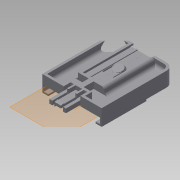
# Autodesk Inventor part: Wanne
Saved by Autodesk Inventor 2015 (Build 190159000, 159)
## iProperties
Created: 2016-03-30
Part Number: Wanne
Material: Generisch
Document SubType Name: Modeling
Designer: Bene
Density: 1 g/cm^3
Appearance: Vorgabe
Author: Bene
Autodesk Inventor part; units mm, degrees
ref_plane "YZ Plane" through (0, 0, 0) normal (1, 0, 0) x (0, 1, 0)
ref_plane "XZ Plane" through (0, 0, 0) normal (0, 1, 0) x (-1, 0, 0)
sketch "Skizze1" plane through (0, 0, 0) normal (0, 0, 1) x (1, 0, 0)
  spline S0 degree 3 poles (-32.4027, 58.6038) (-32.4242, 58.2127) (-32.4349, 57.8189) (-32.4464, 57.0431) (-32.4479, 56.5998) (-32.4483, 56.24) knots 0 0 0 0 0.502492 0.502492 1 1 1 1
  spline S1 degree 3 poles (-20.1386, 68.0766) (-22.3806, 68.0766) (-24.2323, 68.0757) (-27.4543, 67.1708) (-28.3503, 66.6459) (-29.5894, 65.7879) (-30.2592, 65.1575) (-31.2004, 63.6796) (-31.6677, 62.8135) (-32.3154, 60.3747) (-32.41, 59.3008) (-32.4496, 58.5318) knots 0 0 0 0 0.672578 0.672578 1.163557 1.163557 1.787429 1.787429 2.153382 2.153382 2.479485 2.479485 2.479485 2.479485
  line L0 (20.1262, 68.08) -> (-20.1416, 68.08)
  spline S2 degree 3 poles (32.4493, 58.5386) (32.4116, 59.2663) (32.3242, 60.2689) (31.7597, 62.5356) (31.3605, 63.3619) (30.4007, 65.0232) (29.6947, 65.6721) (28.4754, 66.5948) (27.6054, 67.0699) (24.5181, 68.0769) (22.4773, 68.0766) (20.1224, 68.0766) knots 0 0 0 0 0.218603 0.218603 0.458625 0.458625 0.933122 0.933122 1.531383 1.531383 2.646416 2.646416 2.646416 2.646416
  spline S3 degree 3 poles (32.4483, 56.2387) (32.4479, 56.5985) (32.4464, 57.0427) (32.435, 57.8141) (32.4245, 58.2022) (32.4036, 58.5883) knots 0 0 0 0 0.500631 0.500631 1 1 1 1
  line L1 (32.4484, 56.24) -> (32.4914, 56.24)
  spline S4 degree 3 poles (32.4916, 55.7088) (32.4916, 55.8023) (32.4916, 55.8867) (32.4915, 56.0637) (32.4915, 56.1519) (32.4914, 56.24) knots 0 0 0 0 0.502221 0.502221 1 1 1 1
  line L2 (32.495, -55.7116) -> (32.495, 55.7118)
  spline S5 degree 3 poles (32.4914, -56.24) (32.4915, -56.1518) (32.4915, -56.0635) (32.4916, -55.8863) (32.4916, -55.7993) (32.4916, -55.7082) knots 0 0 0 0 0.497816 0.497816 1 1 1 1
  line L3 (32.4483, -56.24) -> (32.4914, -56.24)
  spline S6 degree 3 poles (32.4036, -58.5883) (32.4245, -58.2023) (32.435, -57.8137) (32.4464, -57.0431) (32.4479, -56.5998) (32.4483, -56.24) knots 0 0 0 0 0.499187 0.499187 1 1 1 1
  spline S7 degree 3 poles (20.1238, -68.0766) (22.37, -68.0766) (24.2191, -68.0767) (27.4415, -67.1764) (28.3392, -66.6524) (29.5878, -65.7904) (30.256, -65.1597) (31.1955, -63.6888) (31.6649, -62.8216) (32.3151, -60.3783) (32.4099, -59.3023) (32.4496, -58.5321) knots 0 0 0 0 0.673858 0.673858 1.166886 1.166886 1.797679 1.797679 2.170612 2.170612 2.502894 2.502894 2.502894 2.502894
  line L4 (-20.1262, -68.08) -> (20.1267, -68.08)
  spline S8 degree 3 poles (-32.4488, -58.5488) (-32.4087, -59.3142) (-32.3134, -60.3877) (-31.6647, -62.8189) (-31.1986, -63.684) (-30.2648, -65.1459) (-29.6029, -65.78) (-28.3413, -66.651) (-27.4446, -67.175) (-24.2213, -68.0768) (-22.3702, -68.0766) (-20.1233, -68.0766) knots 0 0 0 0 0.22994 0.22994 0.486349 0.486349 0.910106 0.910106 1.233054 1.233054 1.675094 1.675094 1.675094 1.675094
  spline S9 degree 3 poles (-32.4483, -56.2387) (-32.4479, -56.5985) (-32.4464, -57.0427) (-32.435, -57.8141) (-32.4245, -58.2022) (-32.4036, -58.5883) knots 0 0 0 0 0.500631 0.500631 1 1 1 1
  line L5 (-32.4484, -56.24) -> (-32.4914, -56.24)
  spline S10 degree 3 poles (-32.4916, -55.7088) (-32.4916, -55.8023) (-32.4916, -55.8867) (-32.4915, -56.0637) (-32.4915, -56.1519) (-32.4914, -56.24) knots 0 0 0 0 0.502221 0.502221 1 1 1 1
  line L6 (-32.495, 55.7116) -> (-32.495, -55.7118)
  spline S11 degree 3 poles (-32.4914, 56.24) (-32.4915, 56.1518) (-32.4915, 56.0635) (-32.4916, 55.8863) (-32.4916, 55.7993) (-32.4916, 55.7082) knots 0 0 0 0 0.497816 0.497816 1 1 1 1
  line L7 (-32.4483, 56.24) -> (-32.4914, 56.24)
  line L8 (11, -17.58) -> (-11, -17.58)
  line L9 (-11, -17.58) -> (-11, -68.08)
  line L10 (-11, -68.08) -> (11, -68.08)
  line L11 (11, -68.08) -> (11, -17.58)
  line L12 (0, -17.58) -> (36.495, -17.58)
  line L13 (36.495, -17.58) -> (36.495, 62.08)
  line L14 (27.495, 71.08) -> (0, 71.08)
  line L15 (0, 71.08) -> (0, -17.58)
  line L16 (20.1263, 68.08) -> (-20.1435, 68.08)
  arc A0 (36.495, 62.08) -> (27.495, 71.08) centre (27.495, 62.08) ccw
  line L17 (-0.0077, 79.9624) -> (-0.0077, -73.7985)
  line L18 (-20.1416, 68.08) -> (20.1262, 68.08)
  spline S12 degree 3 poles (-32.4646, 58.5386) (-32.4269, 59.2663) (-32.3395, 60.2689) (-31.775, 62.5356) (-31.3758, 63.3619) (-30.416, 65.0232) (-29.7101, 65.6721) (-28.4907, 66.5948) (-27.6207, 67.0699) (-24.5335, 68.0769) (-22.4926, 68.0766) (-20.1378, 68.0766) knots 0 0 0 0 0.218603 0.218603 0.458625 0.458625 0.933122 0.933122 1.531383 1.531383 2.646416 2.646416 2.646416 2.646416
  spline S13 degree 3 poles (-32.4637, 56.2387) (-32.4633, 56.5985) (-32.4618, 57.0427) (-32.4504, 57.8141) (-32.4399, 58.2022) (-32.4189, 58.5883) knots 0 0 0 0 0.500631 0.500631 1 1 1 1
  line L19 (-32.4638, 56.24) -> (-32.5067, 56.24)
  spline S14 degree 3 poles (-32.5069, 55.7088) (-32.5069, 55.8023) (-32.5069, 55.8867) (-32.5069, 56.0637) (-32.5068, 56.1519) (-32.5067, 56.24) knots 0 0 0 0 0.502221 0.502221 1 1 1 1
  line L20 (-32.5104, -55.7116) -> (-32.5104, 55.7118)
  line L21 (-11.0154, -17.58) -> (10.9846, -17.58)
  line L22 (-11.0154, -68.08) -> (-11.0154, -17.58)
  line L23 (-0.0154, -17.58) -> (-36.5104, -17.58)
  line L24 (-36.5104, -17.58) -> (-36.5104, 62.08)
  line L25 (-27.5104, 71.08) -> (-0.0154, 71.08)
  line L26 (-0.0154, 71.08) -> (-0.0154, -17.58)
  line L27 (-20.1417, 68.08) -> (20.1281, 68.08)
  arc A1 (-27.5104, 71.08) -> (-36.5104, 62.08) centre (-27.5104, 62.08) ccw
  point P0 (0, 0)
  point P1 (-0.0154, 0)
  dimension "d0" = 3
  dimension "d1" = 4
  dimension "d2" = 9
  constraints: 22 symmetric about line, 18 end point, 4 point on circle, 2 centre point, 2 parallel, 2 tangent, 1 horizontal, 1 midpoint, 1 perpendicular, 1 vertical, 1 other
  measures "d0" distance between parallel lines of L14 L16
  measures "d1" distance between parallel lines of L13 L2
  measures "d2" radius of A0
extrude "Extrusion1" add sketch "Skizze1" along normal blind 3 contours L15 L14 A0 L13 L12 L8 | L26 L8 L21 L23 L24 A1 L25
ref_plane "Arbeitsebene1" through (0, 0, 0) normal (0, 0, 1) x (1, 0, 0)
ref_plane "Arbeitsebene2" through (-10.5, -17.58, 1.25) normal (0, 0, 1) x (1, 0, 0)
sketch "Skizze2" plane through (-10.5, -17.58, 1.25) normal (0, 0, 1) x (1, 0, 0)
  line L0 (21.5, 0) -> (-0.5, 0) projected
  line L1 (-0.5, 0) -> (-0.5, -50.5) projected
  line L2 (-0.5, -50.5) -> (21.5, -50.5) projected
  line L3 (21.5, -50.5) -> (21.5, 0) projected
  line L4 (0, 0) -> (21, 0) projected
  line L5 (0, 0) -> (0, -17.5) projected
  line L6 (0, -17.5) -> (21, -17.5) projected
  line L7 (21, 0) -> (21, -17.5) projected
  line L8 (20.6414, -17.5) -> (16.6414, -17.5)
  line L9 (16.6414, -17.5) -> (16.6414, 8.5)
  line L10 (16.6414, 8.5) -> (20.6414, 8.5)
  line L11 (20.6414, 8.5) -> (20.6414, -17.5)
  line L12 (10.5, -17.5) -> (14.5, -17.5)
  line L13 (14.5, -17.5) -> (14.5, 8.5)
  line L14 (14.5, 8.5) -> (10.5, 8.5)
  line L15 (10.5, 8.5) -> (10.5, -17.5)
  line L16 (10.5, -21.3506) -> (10.5, 17.58)
  line L17 (-0.5, 0) -> (21.5, 0)
  line L18 (21, 0) -> (0, 0)
  line L19 (0, 0) -> (0, -17.5)
  line L20 (0.3587, -17.5) -> (4.3587, -17.5)
  line L21 (4.3587, -17.5) -> (4.3587, 8.5)
  line L22 (4.3587, 8.5) -> (0.3587, 8.5)
  line L23 (0.3587, 8.5) -> (0.3587, -17.5)
  line L24 (10.5, -17.5) -> (6.5, -17.5)
  line L25 (6.5, -17.5) -> (6.5, 8.5)
  line L26 (6.5, 8.5) -> (10.5, 8.5)
  line L27 (10.5, 8.5) -> (10.5, -17.5)
  dimension "d5" = 4
  dimension "d6" = 26
  dimension "d7" = 4
  constraints: 34 end point, 13 symmetric about line, 4 parallel, 3 point on line, 2 horizontal, 2 perpendicular, 1 midpoint, 1 vertical
  measures "d5" distance of L9.end L10.end
  measures "d6" distance of L8.end L9.end
  measures "d7" distance of L14.end L13.end
extrude "Extrusion2" add sketch "Skizze2" along normal blind 5 contours L11 L6 L9 L0 | L0 L9 L10 L11 | L13 L6 L15 L0 | L0 L15 L14 L13 | L15 L6 L25 L0 | L0 L25 L26 L15 | L23 L22 L21 L0 | L0 L21 L6 L23
sketch "Skizze3" plane through (4, -35.08, 1.25) normal (1, 0, 0) x (0, 0, -1)
  line L0 (-1.75, 26) -> (-1.75, 17.5) projected
  line L1 (-1.75, 26) -> (-5, 26) projected
  line L2 (-5, 0) -> (-5, 26) projected
  line L3 (0, 0) -> (-5, 0) projected
  line L4 (0, 0) -> (0, 17.5) projected
  line L5 (-1.75, 17.5) -> (0, 17.5) projected
  line L6 (-5, 0) -> (-5.747, 3.8675)
  line L7 (-5.747, 3.8675) -> (-5, 3.8675)
  point P0 (1.25, 35.08)
  constraints: 4 end point, 1 perpendicular, 1 point on line
extrude "Extrusion3" add sketch "Skizze3" against normal up to surface (8 mm away) contours L2 L6 L7
sketch "Skizze4" plane through (-4, -35.08, 1.25) normal (0, -1, 0) x (1, 0, 0)
  line L0 (-6.5, 0) -> (14.5, 0) projected
  line L1 (-6.5, 5.5) -> (-6.5, 0) projected
  line L2 (14.5, 5.5) -> (-6.5, 5.5) projected
  line L3 (14.5, 0) -> (14.5, 5.5) projected
  line L4 (8, 0) -> (8, 5) projected
  line L5 (0.1003, 0) -> (8, 0)
  line L6 (8, 0) -> (8, 1.8913)
  line L7 (8, 1.8913) -> (0.1003, 1.8913)
  line L8 (0.1003, 1.8913) -> (0.1003, 0)
  point P0 (4, -1.25)
  constraints: 8 end point, 2 parallel, 2 point on line, 1 horizontal, 1 perpendicular
extrude "Extrusion4" cut sketch "Skizze4" against normal up to surface (17.5 mm away) contours L8 L7 L4 L0
ref_plane "Arbeitsebene3" through (-29.2488, -52.025, -6.9) normal (0, 0, -1) x (0, 1, 0)
sketch "Skizze5" plane through (0, 0, 0) normal (0, 0, -1) x (-1, 0, 0)
  line L0 (36.5104, -17.58) -> (0.0154, -17.58) projected
  line L1 (36.5104, 62.08) -> (36.5104, -17.58) projected
  arc A0 (36.5104, 62.08) -> (27.5104, 71.08) centre (27.5104, 62.08) ccw projected
  line L2 (0.0154, 71.08) -> (27.5104, 71.08) projected
  line L3 (0.0154, -17.58) -> (0.0154, 71.08) projected
  line L4 (0, -17.58) -> (-36.495, -17.58) projected
  line L5 (0, 71.08) -> (0, -17.58) projected
  line L6 (-27.495, 71.08) -> (0, 71.08) projected
  arc A1 (-27.495, 71.08) -> (-36.495, 62.08) centre (-27.495, 62.08) ccw projected
  line L7 (-36.495, -17.58) -> (-36.495, 62.08) projected
  line L8 (34.6104, -15.68) -> (1.9154, -15.68)
  line L9 (1.9154, -15.68) -> (1.9154, 69.18)
  line L10 (1.9154, 69.18) -> (27.5104, 69.18)
  arc A2 (34.6104, 62.08) -> (27.5104, 69.18) centre (27.5104, 62.08) ccw
  line L11 (34.6104, 62.08) -> (34.6104, -15.68)
  arc A3 (-27.495, 69.18) -> (-34.595, 62.08) centre (-27.495, 62.08) ccw
  line L12 (-27.495, 69.18) -> (-1.9, 69.18)
  line L13 (-1.9, 69.18) -> (-1.9, -15.68)
  line L14 (-1.9, -15.68) -> (-34.595, -15.68)
  line L15 (-34.595, -15.68) -> (-34.595, 62.08)
  line L16 (1.9154, -15.68) -> (-1.9, -15.68)
  line L17 (1.9154, 69.18) -> (-1.9, 69.18)
  line L18 (34.6104, -15.68) -> (34.6104, -17.58)
  line L19 (-34.595, -15.68) -> (-34.595, -17.58)
  point P0 (0, 0)
  dimension "d14" = 1.9
  dimension "d15" = 1.9
  constraints: 24 end point, 8 coincident, 4 point on circle, 2 centre point, 2 point on line, 1 parallel, 1 perpendicular, 8 other
  measures "d14" distance between parallel lines of L1 L11
  measures "d15" distance between parallel lines of L7 L15
extrude "Extrusion5" add sketch "Skizze5" along normal up to surface (6.9 mm away) contours L0 L18 L11 A2 L10 L17 L3 L2 A0 L1 | L0 L3 L16 L8 L18 | L3 L17 L9 L16 | L16 L13 L17 L5 | L5 L4 L19 L14 L16 | L17 L12 A3 L15 L19 L4 L7 A1 L6 L5
sketch "Skizze6" plane through (36.495, -17.58, -6.9) normal (0, 0, -1) x (-1, 0, 0)
  line L0 (38.4104, 1.9) -> (71.1054, 1.9) projected
  line L1 (38.4104, 86.76) -> (38.4104, 1.9) projected
  line L2 (64.0054, 86.76) -> (38.4104, 86.76) projected
  arc A0 (71.1054, 79.66) -> (64.0054, 86.76) centre (64.0054, 79.66) ccw projected
  line L3 (71.1054, 1.9) -> (71.1054, 79.66) projected
  line L4 (36.5104, 0) -> (36.5104, 88.66) projected
  line L5 (73.0054, 0) -> (36.5104, 0) projected
  line L6 (73.0054, 79.66) -> (73.0054, 0) projected
  arc A1 (73.0054, 79.66) -> (64.0054, 88.66) centre (64.0054, 79.66) ccw projected
  line L7 (36.5104, 88.66) -> (64.0054, 88.66) projected
  line L8 (0, 0) -> (0, 79.66) projected
  line L9 (36.495, 0) -> (0, 0) projected
  line L10 (36.495, 88.66) -> (36.495, 0) projected
  line L11 (9, 88.66) -> (36.495, 88.66) projected
  arc A2 (9, 88.66) -> (0, 79.66) centre (9, 79.66) ccw projected
  line L12 (1.9, 1.9) -> (34.595, 1.9) projected
  line L13 (1.9, 79.66) -> (1.9, 1.9) projected
  arc A3 (9, 86.76) -> (1.9, 79.66) centre (9, 79.66) ccw projected
  line L14 (34.595, 86.76) -> (9, 86.76) projected
  line L15 (34.595, 1.9) -> (34.595, 86.76) projected
  line L16 (73.0054, 0) -> (46.6364, 0) projected
  line L17 (71.1054, 0) -> (1.9, 0)
  line L18 (1.9, 0) -> (1.9, 76.76)
  line L19 (11.9, 86.76) -> (61.1054, 86.76)
  line L20 (71.1054, 76.76) -> (71.1054, 0)
  arc A4 (71.1054, 76.76) -> (61.1054, 86.76) centre (61.1054, 76.76) ccw
  arc A5 (11.9, 86.76) -> (1.9, 76.76) centre (11.9, 76.76) ccw
  point P0 (36.495, 17.58)
  dimension "d18" = 10
  constraints: 8 end point, 4 point on circle, 4 tangent, 2 centre point, 2 parallel, 1 equal radius, 1 horizontal, 1 perpendicular, 1 point on line
  measures "d18" radius of A4
extrude "Extrusion6" cut sketch "Skizze6" against normal up to surface (6.9 mm away) contours L1 L2 A4 L3 L0 | L0 L20 L5 L4 L19 L1 | A4 L2 A0 L3 | L4 L17 L10 L19 | L10 L9 L18 L12 L15 L19 | L15 L12 L13 A5 L14
sketch "Skizze7" plane through (-0.0154, 71.08, -6.9) normal (0, 0, -1) x (-1, 0, 0)
  line L0 (34.595, -9) -> (34.595, -88.66) projected
  line L1 (34.595, -9) -> (34.595, -88.66) projected
  line L2 (36.495, -88.66) -> (34.595, -88.66) projected
  line L3 (36.495, -9) -> (36.495, -88.66) projected
  arc A0 (36.495, -9) -> (27.495, 0) centre (27.495, -9) ccw projected
  line L4 (0, 0) -> (27.495, 0) projected
  line L5 (0, -1.9) -> (0, 0) projected
  line L6 (0, -1.9) -> (27.495, -1.9) projected
  arc A1 (34.595, -9) -> (27.495, -1.9) centre (27.495, -9) ccw projected
  line L7 (-34.6104, -88.66) -> (-34.6104, -9) projected
  arc A2 (-27.5104, -1.9) -> (-34.6104, -9) centre (-27.5104, -9) ccw projected
  line L8 (-0.0153, -1.9) -> (-27.5104, -1.9) projected
  line L9 (-0.0153, 0) -> (-0.0153, -1.9) projected
  line L10 (-27.5104, 0) -> (-0.0153, 0) projected
  arc A3 (-27.5104, 0) -> (-36.5104, -9) centre (-27.5104, -9) ccw projected
  line L11 (-36.5104, -88.66) -> (-36.5104, -9) projected
  line L12 (-34.6104, -88.66) -> (-36.5104, -88.66) projected
  line L13 (36.495, -88.66) -> (28.995, -88.66)
  line L14 (28.995, -88.66) -> (28.995, -33.66)
  line L15 (28.995, -33.66) -> (36.495, -33.66)
  line L16 (36.495, -33.66) -> (36.495, -88.66)
  line L17 (-36.5104, -88.66) -> (-29.0104, -88.66)
  line L18 (-29.0104, -88.66) -> (-29.0104, -33.66)
  line L19 (-29.0104, -33.66) -> (-36.5104, -33.66)
  line L20 (-36.5104, -33.66) -> (-36.5104, -88.66)
  point P0 (-0.0154, -71.08)
  dimension "d21" = 7.5
  dimension "d22" = 55
  dimension "d23" = 7.5
  constraints: 16 end point, 4 parallel, 2 horizontal, 2 perpendicular, 1 point on line
  measures "d21" distance of L14.end L15.end
  measures "d22" distance of L13.end L14.end
  measures "d23" distance of L19.end L18.end
extrude "Extrusion7" add sketch "Skizze7" along normal blind 2 contours L15 L3 L2 L0 | L0 L13 L14 L15 | L12 L11 L19 L7 | L7 L19 L18 L17
sketch "Skizze8" plane through (0, 0, 3) normal (0, 0, 1) x (1, 0, 0)
  line L0 (0, -9.08) -> (4, -9.08) projected
  line L1 (4, -9.08) -> (4, -17.58) projected
  line L2 (4, -17.58) -> (6.1414, -17.58) projected
  line L3 (6.1414, -17.58) -> (6.1414, -9.08) projected
  line L4 (6.1414, -9.08) -> (10.1414, -9.08) projected
  line L5 (10.1414, -9.08) -> (10.1414, -17.58) projected
  line L6 (10.1414, -17.58) -> (36.495, -17.58) projected
  line L7 (36.495, -17.58) -> (36.495, 62.08) projected
  arc A0 (36.495, 62.08) -> (27.495, 71.08) centre (27.495, 62.08) ccw projected
  line L8 (27.495, 71.08) -> (0, 71.08) projected
  line L9 (0, 71.08) -> (0, -9.08) projected
  line L10 (-10.1414, -17.58) -> (-10.1414, -9.08) projected
  line L11 (-10.1414, -9.08) -> (-6.1414, -9.08) projected
  line L12 (-6.1414, -9.08) -> (-6.1414, -17.58) projected
  line L13 (-6.1414, -17.58) -> (-4, -17.58) projected
  line L14 (-4, -17.58) -> (-4, -9.08) projected
  line L15 (-4, -9.08) -> (-0.0154, -9.08) projected
  line L16 (-0.0154, -9.08) -> (-0.0154, 71.08) projected
  line L17 (-0.0154, 71.08) -> (-27.5104, 71.08) projected
  arc A1 (-27.5104, 71.08) -> (-36.5104, 62.08) centre (-27.5104, 62.08) ccw projected
  line L18 (-36.5104, 62.08) -> (-36.5104, -17.58) projected
  line L19 (-36.5104, -17.58) -> (-10.1414, -17.58) projected
  point P0 (0, 0)
extrude "Extrusion8" add sketch "Skizze8" along normal blind 8
sketch "Skizze9" plane through (-27.5104, 71.08, -6.9) normal (0, 1, 0) x (1, 0, 0)
  line L0 (27.5104, 0) -> (27.5104, -17.9) projected
  line L1 (55.0054, -17.9) -> (27.5104, -17.9) projected
  line L2 (55.0054, 0) -> (55.0054, -17.9) projected
  line L3 (55.0054, 0) -> (27.5104, 0) projected
  line L4 (0, 0) -> (0, -17.9) projected
  line L5 (27.495, -17.9) -> (0, -17.9) projected
  line L6 (27.495, 0) -> (27.495, -17.9) projected
  line L7 (27.495, 0) -> (0, 0) projected
  line L8 (27.495, -15.9) -> (42.995, -15.9)
  line L9 (42.995, -15.9) -> (42.995, -13.1)
  line L10 (42.995, -13.1) -> (27.495, -13.1)
  line L11 (27.495, -13.1) -> (27.495, -15.9)
  line L12 (27.495, -17.9) -> (40.745, -17.9)
  line L13 (40.745, -17.9) -> (40.745, -15.9)
  line L14 (40.745, -15.9) -> (27.495, -15.9)
  line L15 (27.495, -15.9) -> (27.495, -17.9)
  line L16 (27.5257, -15.9) -> (12.0257, -15.9)
  line L17 (12.0257, -15.9) -> (12.0257, -13.1)
  line L18 (12.0257, -13.1) -> (27.5257, -13.1)
  line L19 (27.5257, -13.1) -> (27.5257, -15.9)
  line L20 (27.5257, -17.9) -> (14.2757, -17.9)
  line L21 (14.2757, -17.9) -> (14.2757, -15.9)
  line L22 (14.2757, -15.9) -> (27.5257, -15.9)
  line L23 (27.5257, -15.9) -> (27.5257, -17.9)
  point P0 (27.5104, -6.9)
  dimension "d28" = 15.5
  dimension "d29" = 2.8
  dimension "d30" = 2
  dimension "d31" = 13.25
  constraints: 32 end point, 8 symmetric about line, 4 parallel, 3 point on line, 2 horizontal, 2 perpendicular
  measures "d28" distance of L10.end L9.end
  measures "d29" distance of L9.end L8.end
  measures "d30" distance between parallel lines of L8 L1
  measures "d31" distance of L14.end L13.end
extrude "Extrusion9" cut sketch "Skizze9" against normal blind 62 contours L10 L19 L8 L0 | L0 L8 L6 L10 | L8 L23 L1 L0 | L0 L12 L6 L8 | L10 L9 L8 L19 | L6 L16 L17 L18 | L6 L5 L21 L16 | L8 L13 L1 L23
sketch "Skizze10" plane through (0, 9.08, 6.2) normal (0, 0, 1) x (1, 0, 0)
  line L0 (0, 0) -> (0, 62) projected
  line L1 (0, 0) -> (15.4847, 0) projected
  line L2 (15.4847, 62) -> (15.4847, 0) projected
  line L3 (0, 62) -> (15.4847, 62) projected
  line L4 (-0.0153, 62) -> (-0.0153, 0) projected
  line L5 (-15.4847, 62) -> (-0.0153, 62) projected
  line L6 (-15.4847, 62) -> (-15.4847, 0) projected
  line L7 (-15.4847, 0) -> (-0.0153, 0) projected
  line L8 (-0.0153, 6) -> (-0.0153, 30) construction
  line L9 (-0.0153, 62) -> (-0.0153, 0) projected
  line L10 (5.6514, 6) -> (5.6514, 30)
  line L11 (-5.6821, 30) -> (-5.6821, 6)
  arc A0 (-5.6821, 6) -> (5.6514, 6) centre (-0.0153, 6) ccw
  arc A1 (5.6514, 30) -> (-5.6821, 30) centre (-0.0153, 30) ccw
  line L12 (-0.0153, 6) -> (-0.0153, 30) construction
  line L13 (7.2771, 6) -> (7.2771, 30)
  line L14 (-7.3077, 30) -> (-7.3077, 6)
  arc A2 (-7.3077, 6) -> (7.2771, 6) centre (-0.0153, 6) ccw
  arc A3 (7.2771, 30) -> (-7.3077, 30) centre (-0.0153, 30) ccw
  line L15 (7.2771, 18) -> (-7.3077, 18)
  point P0 (0, -9.08)
  point P1 (-0.0153, 18)
  point P2 (5.6514, 18)
  point P3 (-5.6821, 18)
  dimension "d34" = 30
  dimension "d35" = 18
  constraints: 18 end point, 8 point on circle, 8 tangent, 6 midpoint, 4 centre point, 4 point on line, 3 parallel, 2 coincident
  measures "d34" distance of L4.end L8.end
  measures "d35" distance between parallel lines of L15 L1
extrude "Extrusion10" cut sketch "Skizze10" against normal blind 32 contours A1 L4 A3 L0 | L0 A3 L13 L15 L10 A1 | A1 L11 L15 L14 A3 L4
sketch "Skizze11" plane through (-15.4847, 71.08, 6.2) normal (0, 0, 1) x (1, 0, 0)
  arc A0 (22.7617, -32) -> (15.4847, -24.7076) centre (15.4693, -32) ccw projected
  line L0 (22.7617, -32) -> (22.7617, -44) projected
  line L1 (22.7617, -44) -> (21.1361, -44) projected
  line L2 (21.1361, -44) -> (21.1361, -32) projected
  arc A1 (21.1361, -32) -> (15.4847, -26.3332) centre (15.4693, -32) ccw projected
  line L3 (15.4847, -62) -> (15.4847, -26.3332) projected
  line L4 (15.4847, -62) -> (30.9693, -62) projected
  line L5 (30.9693, 0) -> (30.9693, -62) projected
  line L6 (15.4847, 0) -> (30.9693, 0) projected
  line L7 (15.4847, -24.7076) -> (15.4847, 0) projected
  arc A2 (15.4693, -26.3332) -> (9.8025, -32) centre (15.4693, -32) ccw projected
  line L8 (9.8025, -32) -> (9.8025, -44) projected
  line L9 (9.8025, -44) -> (8.1769, -44) projected
  line L10 (8.1769, -44) -> (8.1769, -32) projected
  arc A3 (15.4693, -24.7076) -> (8.1769, -32) centre (15.4693, -32) ccw projected
  line L11 (15.4693, 0) -> (15.4693, -24.7076) projected
  line L12 (0, 0) -> (15.4693, 0) projected
  line L13 (0, 0) -> (0, -62) projected
  line L14 (0, -62) -> (15.4693, -62) projected
  line L15 (15.4693, -26.3332) -> (15.4693, -62) projected
  circle A4 centre (15.4693, -32) radius 5.6668
  point P0 (15.4847, -71.08)
  constraints: 1 centre point, 1 coincident, 1 concentric
extrude "Extrusion11" add sketch "Skizze11" along normal blind 2 contours A4 L3 A1 | L3 A4 L15 | L15 A4 A2
sketch "Skizze12" plane through (-0.0154, -17.58, 1.25) normal (1, 0, 0) x (0, 0, -1)
  line L0 (-6.95, 62.3268) -> (-6.95, 50.9932) projected
  line L1 (1.25, 56.66) -> (1.25, 62.3268) projected
  line L2 (-4.95, 56.66) -> (1.25, 56.66) projected
  line L3 (-4.95, 50.9932) -> (-4.95, 56.66) projected
  line L4 (-4.95, 50.9932) -> (-4.95, 50.9932) projected
  line L5 (-4.95, 56.66) -> (-4.95, 50.9932) projected
  line L6 (-4.95, 56.66) -> (1.25, 56.66) projected
  line L7 (1.25, 62.3268) -> (1.25, 56.66) projected
  line L8 (-4.95, 62.3268) -> (1.25, 62.3268) projected
  line L9 (-4.95, 62.3268) -> (-4.95, 62.3268) projected
  line L10 (1.25, 62.3268) -> (-4.95, 62.3268) projected
  line L11 (-4.95, 50.9932) -> (-6.95, 62.3268)
  line L12 (-6.95, 62.3268) -> (-11.4437, 61.5338)
  line L13 (-11.4437, 61.5338) -> (-9.4437, 50.2002)
  line L14 (-9.4437, 50.2002) -> (-4.95, 50.9932)
  point P0 (1.25, 17.58)
  constraints: 8 end point, 2 parallel, 1 perpendicular
extrude "Extrusion12" cut sketch "Skizze12" along normal mid plane 16
sketch "Skizze13" plane through (0, 9.08, 6.2) normal (0, 0, 1) x (1, 0, 0)
  line L0 (-29.25, 42.945) -> (29.25, 42.945) projected
  line L1 (0, 0) -> (0, 24.3332) projected
  line L2 (0, 0) -> (15.4847, 0) projected
  line L3 (15.4847, 62) -> (15.4847, 0) projected
  line L4 (0, 62) -> (15.4847, 62) projected
  line L5 (0, 37.2924) -> (0, 62) projected
  arc A0 (7.2771, 30) -> (0, 37.2924) centre (-0.0153, 30) ccw projected
  line L6 (7.2771, 30) -> (7.2771, 18) projected
  line L7 (7.2771, 18) -> (5.6514, 18) projected
  line L8 (5.6514, 18) -> (5.6514, 30) projected
  arc A1 (0, 24.3332) -> (5.6514, 30) centre (-0.0153, 30) ccw projected
  line L9 (-5.6821, 30) -> (-5.6821, 18) projected
  line L10 (-5.6821, 18) -> (-7.3077, 18) projected
  line L11 (-7.3077, 18) -> (-7.3077, 30) projected
  arc A2 (-0.0153, 37.2924) -> (-7.3077, 30) centre (-0.0153, 30) ccw projected
  line L12 (-0.0153, 62) -> (-0.0153, 37.2924) projected
  line L13 (-15.4847, 62) -> (-0.0153, 62) projected
  line L14 (-15.4847, 62) -> (-15.4847, 0) projected
  line L15 (-15.4847, 0) -> (-0.0153, 0) projected
  line L16 (-0.0153, 24.3332) -> (-0.0153, 0) projected
  arc A3 (-5.6821, 30) -> (-0.0153, 24.3332) centre (-0.0153, 30) ccw projected
  line L17 (0, 62) -> (15.4847, 62) projected
  line L18 (7.6771, 0) -> (7.6771, 62)
  line L19 (7.6771, 62) -> (9.6771, 62)
  line L20 (9.6771, 62) -> (9.6771, 0)
  line L21 (9.6771, 0) -> (7.6771, 0)
  line L22 (-7.75, 0) -> (-7.75, 62)
  line L23 (-7.75, 62) -> (-9.75, 62)
  line L24 (-9.75, 62) -> (-9.75, 0)
  line L25 (-9.75, 0) -> (-7.75, 0)
  point P0 (0, -9.08)
  dimension "d42" = 2
  dimension "d43" = 2
  dimension "d45" = 0.4422
  dimension "d46" = 0.4
  constraints: 16 end point, 4 parallel, 3 perpendicular, 2 midpoint, 2 point on line
  measures "d42" distance of L18.end L19.end
  measures "d43" distance of L23.end L22.end
  measures "d45" distance between parallel lines of L11 L22
  measures "d46" distance between parallel lines of L18 L6
extrude "Extrusion13" add sketch "Skizze13" along normal blind 1 contours L24 L13 L22 L0 | L0 L22 L15 L24 | L18 L4 L20 L0 | L0 L20 L2 L18
sketch "Skizze14" plane through (-10.5, -17.58, 6.25) normal (0, 0, 1) x (1, 0, 0)
  line L0 (21.5, 0) -> (-0.5, 0) projected
  line L1 (-0.5, 0) -> (-0.5, -50.5) projected
  line L2 (-0.5, -50.5) -> (21.5, -50.5) projected
  line L3 (21.5, -50.5) -> (21.5, 0) projected
  line L4 (14.5, -13.6325) -> (14.5, -17.5) projected
  line L5 (14.5, -13.6325) -> (6.5, -13.6325) projected
  line L6 (6.5, -13.6325) -> (6.5, -17.5) projected
  line L7 (5.8587, -19) -> (5.8587, 0)
  line L8 (5.8587, 0) -> (3.8587, 0)
  line L9 (3.8587, 0) -> (3.8587, -19)
  line L10 (3.8587, -19) -> (5.8587, -19)
  line L11 (4.3587, -19) -> (4.3587, -17.6435) projected
  line L12 (15.1414, -19) -> (15.1414, 0)
  line L13 (15.1414, 0) -> (17.1414, 0)
  line L14 (17.1414, 0) -> (17.1414, -19)
  line L15 (17.1414, -19) -> (15.1414, -19)
  line L16 (6.5, -17.5) -> (14.5, -17.5) projected
  point P0 (10.5, 17.58)
  point P1 (5.8587, -17.6435)
  dimension "d50" = 2
  dimension "d51" = 2
  constraints: 16 end point, 5 parallel, 3 perpendicular, 2 point on line
  measures "d50" distance of L8.end L7.end
  measures "d51" distance of L12.end L13.end
extrude "Extrusion14" cut sketch "Skizze14" along normal mid plane 100 contours L14 L15 L12 L0 | L7 L10 L9 L0
sketch "Skizze15" plane through (-3.8997, -35.08, 1.25) normal (0, -1, 0) x (-1, 0, 0)
  line L0 (-2.2416, 7.738) -> (-2.2416, 0) projected
  line L1 (-2.2416, 0) -> (0, 0) projected
  line L2 (0, 0) -> (0, 1.8913) projected
  line L3 (0, 1.8913) -> (7.0411, 1.8913) projected
  line L4 (7.0411, 1.8913) -> (7.0411, 7.738) projected
  line L5 (-2.2416, 7.738) -> (7.0411, 7.738) projected
  line L6 (6.7416, 1.8913) -> (-2.2416, 1.8913)
  line L7 (-2.2416, 1.8913) -> (-2.2416, 7.738)
  line L8 (-2.2416, 7.738) -> (6.7416, 7.738)
  line L9 (6.7416, 7.738) -> (6.7416, 1.8913)
  point P0 (-3.8997, 1.25)
  constraints: 8 end point, 2 parallel, 2 perpendicular, 2 point on line
extrude "Extrusion15" cut sketch "Skizze15" against normal up to surface (17.5 mm away) contours L6 L2 L1 L0
sketch "Skizze16" plane through (0, 0, 11) normal (0, 0, 1) x (1, 0, 0)
  line L0 (13.2346, 9.08) -> (0, 9.08) projected
  line L1 (0, 9.08) -> (0, -9.08) projected
  line L2 (0, -9.08) -> (4, -9.08) projected
  line L3 (4, -9.08) -> (4, -17.58) projected
  line L4 (4, -17.58) -> (6.1414, -17.58) projected
  line L5 (6.1414, -17.58) -> (6.1414, -9.08) projected
  line L6 (6.1414, -9.08) -> (10.1414, -9.08) projected
  line L7 (10.1414, -9.08) -> (10.1414, -17.58) projected
  line L8 (10.1414, -17.58) -> (36.495, -17.58) projected
  line L9 (36.495, -17.58) -> (36.495, 62.08) projected
  arc A0 (36.495, 62.08) -> (27.495, 71.08) centre (27.495, 62.08) ccw projected
  line L10 (27.495, 71.08) -> (13.2346, 71.08) projected
  line L11 (13.2346, 71.08) -> (13.2346, 9.08) projected
  line L12 (-0.0154, 9.08) -> (-13.2347, 9.08) projected
  line L13 (-13.2347, 9.08) -> (-13.2347, 71.08) projected
  line L14 (-13.2347, 71.08) -> (-27.5104, 71.08) projected
  arc A1 (-27.5104, 71.08) -> (-36.5104, 62.08) centre (-27.5104, 62.08) ccw projected
  line L15 (-36.5104, 62.08) -> (-36.5104, -17.58) projected
  line L16 (-36.5104, -17.58) -> (-10.1414, -17.58) projected
  line L17 (-10.1414, -17.58) -> (-10.1414, -9.08) projected
  line L18 (-10.1414, -9.08) -> (-6.1414, -9.08) projected
  line L19 (-6.1414, -9.08) -> (-6.1414, -17.58) projected
  line L20 (-6.1414, -17.58) -> (-4, -17.58) projected
  line L21 (-4, -17.58) -> (-4, -9.08) projected
  line L22 (-4, -9.08) -> (-0.0154, -9.08) projected
  line L23 (-0.0154, -9.08) -> (-0.0154, 9.08) projected
  line L24 (33.495, -14.58) -> (13.1414, -14.58)
  line L25 (13.1414, -14.58) -> (13.1414, -6.08)
  line L26 (13.1414, -6.08) -> (7, -6.08)
  line L27 (7, -6.08) -> (3, -6.08)
  line L28 (3, -6.08) -> (3, 6.08)
  line L29 (3, 6.08) -> (16.2346, 6.08)
  line L30 (16.2346, 6.08) -> (16.2346, 68.08)
  line L31 (16.2346, 68.08) -> (27.495, 68.08)
  arc A2 (33.495, 62.08) -> (27.495, 68.08) centre (27.495, 62.08) ccw
  line L32 (33.495, 62.08) -> (33.495, -14.58)
  line L33 (-33.5104, -14.58) -> (-33.5104, 62.08)
  arc A3 (-27.5104, 68.08) -> (-33.5104, 62.08) centre (-27.5104, 62.08) ccw
  line L34 (-27.5104, 68.08) -> (-16.2347, 68.08)
  line L35 (-16.2347, 68.08) -> (-16.2347, 6.08)
  line L36 (-16.2347, 6.08) -> (-3.0154, 6.08)
  line L37 (-3.0154, 6.08) -> (-3.0154, -6.08)
  line L38 (-3.0154, -6.08) -> (-3.1414, -6.08)
  line L39 (-3.1414, -6.08) -> (-13.1414, -6.08)
  line L40 (-13.1414, -6.08) -> (-13.1414, -14.58)
  line L41 (-13.1414, -14.58) -> (-33.5104, -14.58)
  point P0 (0, 0)
  dimension "d56" = 3
  dimension "d57" = 3
  constraints: 36 end point, 4 point on circle, 2 centre point, 18 other
  measures "d56" distance between parallel lines of L8 L24
  measures "d57" distance between parallel lines of L15 L33
extrude "Extrusion16" cut sketch "Skizze16" against normal blind 8 contours L24 L25 L26 L27 L28 L29 L30 L31 A2 L32 | L33 A3 L34 L35 L36 L37 L38 L39 L40 L41
fillet "Rundung1" radius 4 9 edges at (31.7376, 66.3226, 3) (21.8648, 68.08, 3) (33.495, 23.75, 3) (-31.753, 66.3226, 3) (-21.8725, 68.08, 3) (-33.5104, 23.75, 3) (16.2346, 37.08, 3) (-16.2347, 37.08, 3) (16.2346, 37.08, 11)
